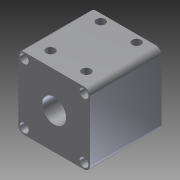
# Autodesk Inventor part: Base
Saved by Autodesk Inventor 2012 SP1 (Build 160190100, 190)
## iProperties
Created: 2012-01-12
Part Number: Base
Material: Default
Document SubType Name: Modeling
Designer: Moses
Density: 1 g/cm^3
Author: Moses
Autodesk Inventor part; units mm, degrees
ref_plane "YZ Plane" through (0, 0, 0) normal (1, 0, 0) x (0, 1, 0)
ref_plane "XZ Plane" through (0, 0, 0) normal (0, 1, 0) x (-1, 0, 0)
ref_plane "XY Plane" through (0, 0, 0) normal (0, 0, 1) x (1, 0, 0)
sketch "Sketch1" plane through (0, 0, 0) normal (0, 0, 1) x (1, 0, 0)
  line L0 (0, 0) -> (0, 38.1)
  line L1 (0, 38.1) -> (38.1, 38.1)
  line L2 (38.1, 38.1) -> (38.1, 0)
  line L3 (38.1, 0) -> (0, 0)
  circle A0 centre (19.05, 19.05) radius 6.35
  circle A1 centre (3.175, 34.925) radius 2.3495
  circle A2 centre (34.925, 34.925) radius 2.3495
  circle A3 centre (3.175, 3.175) radius 2.3495
  circle A4 centre (34.925, 3.175) radius 2.3495
  dimension "d0" = 38.1
  dimension "d1" = 38.1
  dimension "d2" = 12.7
  dimension "d3" = 19.05
  dimension "d4" = 19.05
  dimension "d34" = 4.699
  dimension "d37" = 31.75
  dimension "d40" = 31.75
  dimension "d43" = 3.175
  dimension "d44" = 3.175
  constraints: 8 end point, 5 centre point, 2 perpendicular, 2 vertical, 1 horizontal, 1 parallel, 6 other
  measures "d0" distance of L0.start L0.end
  measures "d1" distance of L0.end L1.end
  measures "d2" diameter of A0
  measures "d3" distance from line of L1 A0.centre
  measures "d4" distance from line of L0 A0.centre
  measures "d34" diameter of A1
  measures "d37" distance of A1.centre A2.centre
  measures "d40" distance of A1.centre A3.centre
  measures "d43" distance from line of L1 A1.centre
  measures "d44" distance from line of L0 A1.centre
extrude "Extrusion1" add sketch "Sketch1" along normal blind 38.1
fillet "Fillet1" radius 3.175 4 edges at (38.1, 38.1, 19.05) (38.1, 0, 19.05) (0, 38.1, 19.05) (0, 0, 19.05)
sketch "Sketch2" plane through (0, 38.1, 0) normal (0, 1, 0) x (1, 0, 0)
  line L0 (0, 0) -> (38.1, 0) projected
  line L1 (0, 0) -> (0, -38.1) projected
  circle A0 centre (9.525, -3.81) radius 2.3495
  circle A1 centre (28.575, -3.81) radius 2.3495
  circle A2 centre (9.525, -30.48) radius 2.3495
  circle A3 centre (28.575, -30.48) radius 2.3495
  dimension "d8" = 4.699
  dimension "d11" = 19.05
  dimension "d14" = 26.67
  dimension "d17" = 3.81
  dimension "d18" = 9.525
  constraints: 4 centre point, 1 horizontal, 1 vertical, 6 other
  measures "d8" diameter of A0
  measures "d11" distance of A0.centre A1.centre
  measures "d14" distance of A0.centre A2.centre
  measures "d17" distance from line of L0 A0.centre
  measures "d18" distance from line of L1 A0.centre
extrude "Extrusion2" cut sketch "Sketch2" against normal blind 7.62
sketch "Sketch3" plane through (0, 0, 0) normal (0, -1, 0) x (1, 0, 0)
  line L0 (38.1, 0) -> (0, 0) projected
  line L1 (38.1, 0) -> (38.1, 38.1) projected
  circle A0 centre (28.575, 3.81) radius 2.3495
  circle A1 centre (9.525, 3.81) radius 2.3495
  circle A2 centre (28.575, 30.48) radius 2.3495
  circle A3 centre (9.525, 30.48) radius 2.3495
  dimension "d21" = 4.699
  dimension "d24" = 19.05
  dimension "d27" = 26.67
  dimension "d30" = 3.81
  dimension "d31" = 9.525
  constraints: 4 centre point, 1 horizontal, 1 vertical, 6 other
  measures "d21" diameter of A0
  measures "d24" distance of A0.centre A1.centre
  measures "d27" distance of A0.centre A2.centre
  measures "d30" distance from line of L0 A0.centre
  measures "d31" distance from line of L1 A0.centre
extrude "Extrusion3" cut sketch "Sketch3" against normal blind 7.62
body "Solid1"
